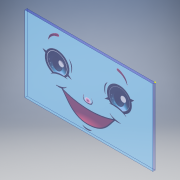
# Autodesk Inventor part: pantalla
Saved by Autodesk Inventor 2019 (Build 230136000, 136)
## iProperties
Created: 2019-02-21
Part Number: pantalla
Material: Genérico
Document SubType Name: Modeling
Designer: flakt
Density: 1 g/cm^3
Appearance: Claro - Azul
Author: flakt
Autodesk Inventor part; units mm, degrees
ref_plane "YZ Plane" through (0, 0, 0) normal (1, 0, 0) x (0, 1, 0)
ref_plane "XZ Plane" through (0, 0, 0) normal (0, 1, 0) x (-1, 0, 0)
ref_plane "XY Plane" through (0, 0, 0) normal (0, 0, 1) x (1, 0, 0)
sketch "Boceto1" plane through (0, 0, 0) normal (0, 0, 1) x (1, 0, 0)
  line L0 (0, 0) -> (113, 0)
  line L1 (113, 0) -> (113, -67)
  line L2 (113, -67) -> (0, -67)
  line L3 (0, -67) -> (0, 0)
  dimension "d0" = 113
  dimension "d1" = 67
  constraints: 8 end point, 2 parallel, 1 horizontal, 1 perpendicular
  measures "d0" distance of L1.end L2.end
  measures "d1" distance of L0.end L1.end
extrude "Extrusión1" add sketch "Boceto1" along normal blind 2
sketch "Boceto2" plane through (0, 0, 2) normal (0, 0, 1) x (1, 0, 0)
  line L0 (113, 0) -> (0, 0) projected
  line L1 (-12.8028, 6.364) -> (124.3271, 6.364) construction
  line L2 (124.3271, 6.364) -> (124.3271, -75.9421) construction
  line L3 (124.3271, -75.9421) -> (-12.8028, -75.9421) construction
  line L4 (-12.8028, -75.9421) -> (-12.8028, 6.364) construction
  constraints: 2 other
sketch "Boceto3" plane through (113, -67, 0) normal (1, 0, 0) x (0, 0, -1)
  point P0 (0, 67)
decal "Calcomanía2"
